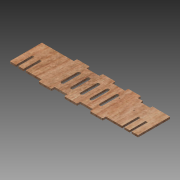
# Autodesk Inventor part: voor-plaat
Saved by Autodesk Inventor 2015 (Build 190159000, 159)
## iProperties
Created: 2015-12-19
Part Number: voor-plaat
Material: Generic
Document SubType Name: Modeling
Designer: david
Density: 1 g/cm^3
Appearance: Birch - Natural Polished
Mass: 28.4153 g
Surface Area: 222.147 cm^2
Volume: 28.4153 cm^3
Author: david
Autodesk Inventor part; units mm, degrees
ref_plane "YZ Plane" through (0, 0, 0) normal (1, 0, 0) x (0, 1, 0)
ref_plane "XZ Plane" through (0, 0, 0) normal (0, 1, 0) x (-1, 0, 0)
ref_plane "XY Plane" through (0, 0, 0) normal (0, 0, 1) x (1, 0, 0)
sketch "Sketch1" plane through (0, 0, 0) normal (0, 0, 1) x (1, 0, 0)
  line L0 (-100, -25) -> (100, -25)
  line L1 (100, -25) -> (100, 25)
  line L2 (100, 25) -> (-100, 25)
  line L3 (-100, 25) -> (-100, -25)
  line L4 (-100, -25) -> (100, 25) construction
  line L5 (100, -25) -> (-100, 25) construction
  point P0 (0, 0)
  dimension "d0" = 200
  dimension "d1" = 50
  constraints: 12 end point, 2 midpoint, 2 parallel, 1 horizontal, 1 perpendicular
  measures "d0" distance of L2.end L1.end
  measures "d1" distance of L1.end L0.end
extrude "Extrusion1" add sketch "Sketch1" along normal blind 3
sketch "Sketch2" plane through (0, 0, 0) normal (0, 0, -1) x (-1, 0, 0)
  line L0 (100, -25) -> (-100, -25) projected
  line L1 (-90.25, -25) -> (-86.75, -25)
  line L2 (-86.75, -25) -> (-86.75, 0)
  line L3 (-86.75, 0) -> (-90.25, 0)
  line L4 (-90.25, 0) -> (-90.25, -25)
  line L5 (86.75, -25) -> (90.25, -25)
  line L6 (90.25, -25) -> (90.25, 0)
  line L7 (90.25, 0) -> (86.75, 0)
  line L8 (86.75, 0) -> (86.75, -25)
  line L9 (-78.75, 0) -> (-75.25, 0)
  line L10 (-75.25, 0) -> (-75.25, -25)
  line L11 (-75.25, -25) -> (-78.75, -25)
  line L12 (-78.75, -25) -> (-78.75, 0)
  line L13 (78.75, 0) -> (75.25, 0)
  line L14 (75.25, 0) -> (75.25, -25)
  line L15 (75.25, -25) -> (78.75, -25)
  line L16 (78.75, -25) -> (78.75, 0)
  point P0 (0, 0)
  dimension "d4" = 3.5
  dimension "d5" = 25
  dimension "d6" = 3.5
  dimension "d7" = 86.75
  dimension "d8" = 86.75
  dimension "d11" = 3.5
  dimension "d12" = 8
  dimension "d13" = 3.5
  dimension "d14" = 8
  constraints: 32 end point, 8 parallel, 5 point on line, 4 horizontal, 4 perpendicular
  measures "d4" distance of L3.end L2.end
  measures "d5" distance of L2.end L1.end
  measures "d6" distance of L7.end L6.end
  measures "d7" distance from line of point (0, 0) L8
  measures "d8" distance from line of L2 point (0, 0)
  measures "d11" distance of L10.end L11.end
  measures "d12" distance between parallel lines of L12 L2
  measures "d13" distance of L15.end L14.end
  measures "d14" distance between parallel lines of L8 L16
extrude "Extrusion2" cut sketch "Sketch2" against normal blind 3
sketch "Sketch3" plane through (0, 0, 3) normal (0, 0, 1) x (1, 0, 0)
  line L0 (-49.25, 30) -> (-31.25, 30)
  line L1 (-30.25, 29) -> (-30.25, -29)
  line L2 (-31.25, -30) -> (-49.25, -30)
  line L3 (-50.25, -29) -> (-50.25, 29)
  line L4 (-50.25, 30) -> (-30.25, -30) construction
  line L5 (-30.25, 30) -> (-50.25, -30) construction
  line L6 (-75.25, -25) -> (75.25, -25) projected
  line L7 (-75.25, 0) -> (-75.25, -25) projected
  arc A0 (-49.25, 30) -> (-50.25, 29) centre (-49.25, 29) ccw
  arc A1 (-30.25, 29) -> (-31.25, 30) centre (-31.25, 29) ccw
  arc A2 (-31.25, -30) -> (-30.25, -29) centre (-31.25, -29) ccw
  arc A3 (-50.25, -29) -> (-49.25, -30) centre (-49.25, -29) ccw
  point P0 (-40.25, 0)
  dimension "d33" = 20
  dimension "d34" = 60
  dimension "d35" = 5
  dimension "d36" = 25
  dimension "d37" = 1
  constraints: 12 end point, 8 point on circle, 8 point on line, 8 tangent, 4 centre point, 3 equal radius, 2 midpoint, 2 parallel, 1 horizontal, 1 perpendicular
  measures "d33" distance of L4.end L5.end
  measures "d34" distance of L5.start L4.end
  measures "d35" distance between parallel lines of L6 L2
  measures "d36" distance between parallel lines of L7 L3
  measures "d37" radius of A0
extrude "Extrusion3" add sketch "Sketch3" against normal blind 3
sketch "Sketch5" plane through (0, 0, 3) normal (0, 0, 1) x (1, 0, 0)
  line L0 (57.5, 21.5) -> (72.5, 21.5)
  line L1 (72.5, 21.5) -> (72.5, 25)
  line L2 (72.5, 25) -> (57.5, 25)
  line L3 (57.5, 25) -> (57.5, 21.5)
  line L4 (57.5, 21.5) -> (72.5, 25) construction
  line L5 (72.5, 21.5) -> (57.5, 25) construction
  line L6 (100, 25) -> (-100, 25) projected
  line L7 (100, -25) -> (100, 25) projected
  point P0 (0, 0)
  point P1 (65, 23.25)
  dimension "d27" = 15
  dimension "d28" = 3.5
  dimension "d29" = 0
  dimension "d38" = 27.5
  constraints: 12 end point, 2 midpoint, 2 parallel, 1 horizontal, 1 perpendicular
  measures "d27" distance of L2.end L1.end
  measures "d28" distance of L1.end L0.end
  measures "d29" distance between parallel lines of L6 L2
  measures "d38" distance between parallel lines of L7 L1
extrude "Extrusion5" cut sketch "Sketch5" against normal blind 10
pattern_linear "Rectangular Pattern2" count 3 spacing 40 along (1, 0, 0) of "Extrusion3"
sketch "Sketch4" plane through (0, 0, 3) normal (0, 0, 1) x (1, 0, 0)
  line L0 (0, 12.5) -> (0, -12.5) construction
  line L1 (-2.5, 12.5) -> (-2.5, -12.5)
  line L2 (2.5, -12.5) -> (2.5, 12.5)
  arc A0 (2.5, 12.5) -> (-2.5, 12.5) centre (0, 12.5) ccw
  arc A1 (-2.5, -12.5) -> (2.5, -12.5) centre (0, -12.5) ccw
  point P0 (0, 0)
  point P1 (0, 0)
  dimension "d19" = 25
  dimension "d20" = 5
  dimension "d21" = 12.5
  constraints: 8 end point, 4 point on circle, 4 tangent, 2 centre point, 1 midpoint, 1 parallel, 1 vertical
  measures "d19" distance of L0.start L0.end
  measures "d20" diameter of A1
  measures "d21" distance of L0.start point (0, 0)
extrude "Extrusion4" cut sketch "Sketch4" against normal blind 4
pattern_linear "Rectangular Pattern1" count 5 spacing 15 along (-1, 0, 0) of "Extrusion4" first direction both ways yes
body "Solid1"
